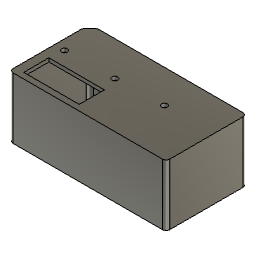
Waterproofing case - PLA case (Autodesk Fusion 360 design; units mm, degrees)
Autodesk Fusion 360 part; units mm, degrees
sketch "Sketch1" plane through (0, 0, 0) normal (0, 0, 1) x (1, 0, 0)
  line L0 (0, 0) -> (104, 0)
  line L1 (104, 0) -> (104, 51)
  line L2 (104, 51) -> (0, 51)
  line L3 (0, 51) -> (0, 0)
  dimension "d1" = 51
  dimension "d2" = 104
  constraint horizontal L0
  constraint vertical L1
  constraint horizontal L2
  constraint vertical L3
  constraint coincident L0.start L3.end
  measures "d1" distance of L0.start L2.end
  measures "d2" distance of L0.start L0.end
extrude "Extrude1" add sketch "Sketch1" along normal blind 2.5
sketch "Sketch2" plane through (0, 0, 2.5) normal (0, 0, 1) x (-1, 0, 0)
  line L0 (0, -51) -> (0, 0)
  line L1 (0, 0) -> (-104, 0)
  line L2 (-104, 0) -> (-104, -51)
  line L3 (-104, -51) -> (0, -51)
  line L4 (2.5, -53.5) -> (-106.5, -53.5)
  line L5 (-106.5, -53.5) -> (-106.5, 2.5)
  line L6 (-106.5, 2.5) -> (2.5, 2.5)
  line L7 (2.5, 2.5) -> (2.5, -53.5)
  dimension "d5" = 2.5
  dimension "d6" = 2.5
  dimension "d7" = 2.5
  dimension "d8" = 2.5
  constraint horizontal L4
  constraint vertical L5
  constraint horizontal L6
  constraint vertical L7
  measures "d5" distance of L1 L6
  measures "d6" distance of L2 L5
  measures "d7" distance of L3 L4
  measures "d8" distance of L0 L7
extrude "Extrude2" add sketch "Sketch2" against normal blind 42.5
fillet "Fillet1" radius 2.5 8 edges at (-2.5, -2.5, -18.75) (106.5, -2.5, -18.75) (106.5, 53.5, -18.75) (0, 0, -20) (-2.5, 53.5, -18.75) (0, 51, -20) (104, 0, -20) (104, 51, -20)
sketch "Sketch3" plane through (0, 0, 0) normal (0, 0, 1) x (1, 0, 0)
  line L0 (100, 19) -> (61.43, 19)
  line L1 (61.43, 19) -> (61.43, 1.5)
  line L2 (61.43, 1.5) -> (100, 1.5)
  line L3 (100, 1.5) -> (100, 19)
  line L4 (2.5, 0) -> (101.5, 0)
  line L5 (104, 2.5) -> (104, 48.5)
  circle A0 centre (97.5, 28.9) radius 2
  circle A1 centre (64.005, 29.5) radius 2
  circle A2 centre (29.495, 30.5) radius 2
  line L6 (106.5, 51) -> (106.5, 0)
  dimension "d13" = 38.57
  dimension "d14" = 17.5
  dimension "d15" = 1.5
  dimension "d16" = 4
  dimension "d17" = 4
  dimension "d18" = 4
  dimension "d19" = 4
  dimension "d20" = 9
  dimension "d21" = 9.9
  dimension "d22" = 10.5
  dimension "d23" = 11.5
  dimension "d24" = 33.495
  dimension "d25" = 34.51
  constraint horizontal L0
  constraint vertical L1
  constraint horizontal L2
  constraint vertical L3
  measures "d13" distance of L0.start L0.end
  measures "d14" distance of L0.start L2.end
  measures "d15" distance of L2 L4
  measures "d16" distance of L3 L5
  measures "d17" diameter of A0
  measures "d18" diameter of A1
  measures "d19" diameter of A2
  measures "d20" distance of A0.centre L6
  measures "d21" distance of L0 A0.centre
  measures "d22" distance of L0 A1.centre
  measures "d23" distance of L0 A2.centre
  measures "d24" horizontal distance of A0.centre A1.centre
  measures "d25" horizontal distance of A1.centre A2.centre
sketch "Sketch7" plane through (0, 0, 2.5) normal (0, 0, 1) x (-1, 0, 0)
  arc A0 (0, -53.5) -> (2.5, -51) centre (0, -51) ccw
  line L0 (2.5, -51) -> (2.5, 0)
  arc A1 (2.5, 0) -> (0, 2.5) centre (0, 0) ccw
  line L1 (0, 2.5) -> (-104, 2.5)
  arc A2 (-104, 2.5) -> (-106.5, 0) centre (-104, 0) ccw
  line L2 (-106.5, 0) -> (-106.5, -51)
  arc A3 (-106.5, -51) -> (-104, -53.5) centre (-104, -51) ccw
  line L3 (-104, -53.5) -> (0, -53.5)
  line L4 (-3.5, -19) -> (-42.07, -19)
  line L5 (-42.07, -19) -> (-42.07, -1.5)
  line L6 (-42.07, -1.5) -> (-3.5, -1.5)
  line L7 (-3.5, -1.5) -> (-3.5, -19)
  circle A4 centre (-6.5, -28.9) radius 2
  circle A5 centre (-41.01, -29.5) radius 2
  circle A6 centre (-74.505, -30.5) radius 2
  dimension "d49" = 38.57
  dimension "d50" = 17.5
  dimension "d51" = 4
  dimension "d52" = 6
  dimension "d53" = 4
  dimension "d54" = 4
  dimension "d55" = 4
  dimension "d56" = 9.9
  dimension "d57" = 10.5
  dimension "d58" = 11.5
  dimension "d59" = 9
  dimension "d60" = 34.51
  dimension "d61" = 33.495
  constraint horizontal L4
  constraint vertical L5
  constraint horizontal L6
  constraint vertical L7
  measures "d49" distance of L4.start L4.end
  measures "d50" distance of L4.start L6.end
  measures "d51" distance of L1 L6
  measures "d52" distance of L0 L7
  measures "d53" diameter of A4
  measures "d54" diameter of A5
  measures "d55" diameter of A6
  measures "d56" distance of L4 A4.centre
  measures "d57" distance of L4 A5.centre
  measures "d58" distance of L4 A6.centre
  measures "d59" distance of L0 A4.centre
  measures "d60" horizontal distance of A4.centre A5.centre
  measures "d61" horizontal distance of A5.centre A6.centre
extrude "Extrude6" cut sketch "Sketch7" against normal blind 50 contours L4 L5 L6 L7 | A4 | A5 | A6
sketch "Sketch8" plane through (0, 0, 0) normal (0, 0, 1) x (1, 0, 0)
sketch "Sketch9" plane through (0, 0, 0) normal (0, 0, -1) x (1, 0, 0)
  circle A0 centre (6.5, -28.9) radius 2
  line L0 (42.07, -1.5) -> (42.07, -19)
  line L1 (42.07, -19) -> (3.5, -19)
  line L2 (3.5, -19) -> (3.5, -1.5)
  line L3 (3.5, -1.5) -> (42.07, -1.5)
  circle A1 centre (41.01, -29.5) radius 2
  circle A2 centre (74.505, -30.5) radius 2
  arc A3 (101.5, -51) -> (104, -48.5) centre (101.5, -48.5) ccw
  line L4 (104, -48.5) -> (104, -2.5)
  arc A4 (104, -2.5) -> (101.5, 0) centre (101.5, -2.5) ccw
  line L5 (101.5, 0) -> (2.5, 0)
  arc A5 (2.5, 0) -> (0, -2.5) centre (2.5, -2.5) ccw
  line L6 (0, -2.5) -> (0, -48.5)
  arc A6 (0, -48.5) -> (2.5, -51) centre (2.5, -48.5) ccw
  line L7 (2.5, -51) -> (101.5, -51)
extrude "Extrude7" add sketch "Sketch9" against normal blind 2.5 contours A0 | A1 | A2
sketch "Sketch10" plane through (0, 0, 0) normal (0, 0, -1) x (1, 0, 0)
  line L0 (42.07, -1.5) -> (42.07, -19)
  line L1 (42.07, -19) -> (3.5, -19)
  line L2 (3.5, -19) -> (3.5, -1.5)
  line L3 (3.5, -1.5) -> (42.07, -1.5)
  arc A0 (101.5, -51) -> (104, -48.5) centre (101.5, -48.5) ccw
  line L4 (104, -48.5) -> (104, -2.5)
  arc A1 (104, -2.5) -> (101.5, 0) centre (101.5, -2.5) ccw
  line L5 (101.5, 0) -> (2.5, 0)
  arc A2 (2.5, 0) -> (0, -2.5) centre (2.5, -2.5) ccw
  line L6 (0, -2.5) -> (0, -48.5)
  arc A3 (0, -48.5) -> (2.5, -51) centre (2.5, -48.5) ccw
  line L7 (2.5, -51) -> (101.5, -51)
  circle A4 centre (4.4, -28.9) radius 2
  circle A5 centre (38.91, -29.5) radius 2
  circle A6 centre (72.405, -30.5) radius 2
  line L8 (0, -48.5) -> (0, -2.5)
  dimension "d66" = 4
  dimension "d67" = 4
  dimension "d68" = 4
  dimension "d69" = 4.4
  dimension "d70" = 38.91
  dimension "d71" = 72.405
  dimension "d72" = 9.9
  dimension "d73" = 10.5
  dimension "d74" = 11.5
  measures "d66" diameter of A4
  measures "d67" diameter of A5
  measures "d68" diameter of A6
  measures "d69" distance of A4.centre L8
  measures "d70" distance of A5.centre L8
  measures "d71" distance of A6.centre L8
  measures "d72" distance of L1 A4.centre
  measures "d73" distance of L1 A5.centre
  measures "d74" distance of L1 A6.centre
extrude "Extrude8" cut sketch "Sketch10" against normal blind 15 contours A4 | A5 | A6
sketch "Sketch11" plane through (0, 0, -40) normal (0, 0, -1) x (1, 0, 0)
  arc A0 (-2.5, -51) -> (0, -53.5) centre (0, -51) ccw
  line L0 (0, -53.5) -> (104, -53.5)
  arc A1 (104, -53.5) -> (106.5, -51) centre (104, -51) ccw
  line L1 (106.5, -51) -> (106.5, 0)
  arc A2 (106.5, 0) -> (104, 2.5) centre (104, 0) ccw
  line L2 (104, 2.5) -> (0, 2.5)
  arc A3 (0, 2.5) -> (-2.5, 0) centre (0, 0) ccw
  line L3 (-2.5, 0) -> (-2.5, -51)
  line L4 (101.5, -51) -> (2.5, -51)
  arc A4 (0, -48.5) -> (2.5, -51) centre (2.5, -48.5) ccw
  line L5 (0, -48.5) -> (0, -2.5)
  arc A5 (2.5, 0) -> (0, -2.5) centre (2.5, -2.5) ccw
  line L6 (2.5, 0) -> (101.5, 0)
  arc A6 (104, -2.5) -> (101.5, 0) centre (101.5, -2.5) ccw
  line L7 (104, -2.5) -> (104, -48.5)
  arc A7 (101.5, -51) -> (104, -48.5) centre (101.5, -48.5) ccw
  line L8 (0, -53.5) -> (-2.5, -51)
  constraint coincident A0.end L0.start
  constraint coincident A0.start L3.end
sketch "Sketch12" plane through (0, 0, -40) normal (0, 0, -1) x (1, 0, 0)
  arc A0 (-2.5, -51) -> (0, -53.5) centre (0, -51) ccw
  line L0 (0, -53.5) -> (104, -53.5)
  arc A1 (104, -53.5) -> (106.5, -51) centre (104, -51) ccw
  line L1 (106.5, -51) -> (106.5, 0)
  arc A2 (106.5, 0) -> (104, 2.5) centre (104, 0) ccw
  line L2 (104, 2.5) -> (0, 2.5)
  arc A3 (0, 2.5) -> (-2.5, 0) centre (0, 0) ccw
  line L3 (-2.5, 0) -> (-2.5, -51)
  line L4 (101.5, -51) -> (2.5, -51)
  arc A4 (0, -48.5) -> (2.5, -51) centre (2.5, -48.5) ccw
  line L5 (0, -48.5) -> (0, -2.5)
  arc A5 (2.5, 0) -> (0, -2.5) centre (2.5, -2.5) ccw
  line L6 (2.5, 0) -> (101.5, 0)
  arc A6 (104, -2.5) -> (101.5, 0) centre (101.5, -2.5) ccw
  line L7 (104, -2.5) -> (104, -48.5)
  arc A7 (101.5, -51) -> (104, -48.5) centre (101.5, -48.5) ccw
  line L8 (0, -53.5) -> (-2.5731, -53.5)
  line L9 (-2.5731, -53.5) -> (-2.5, -51)
  constraint coincident A0.end L0.start
  constraint tangent A0 L8
  constraint coincident A0.start L3.end
sketch "Sketch13" plane through (0, 0, -40) normal (0, 0, -1) x (1, 0, 0)
  arc A0 (-2.5, -51) -> (0, -53.5) centre (0, -51) ccw
  line L0 (0, -53.5) -> (104, -53.5)
  arc A1 (104, -53.5) -> (106.5, -51) centre (104, -51) ccw
  line L1 (106.5, -51) -> (106.5, 0)
  arc A2 (106.5, 0) -> (104, 2.5) centre (104, 0) ccw
  line L2 (104, 2.5) -> (0, 2.5)
  arc A3 (0, 2.5) -> (-2.5, 0) centre (0, 0) ccw
  line L3 (-2.5, 0) -> (-2.5, -51)
  line L4 (101.5, -51) -> (2.5, -51)
  arc A4 (0, -48.5) -> (2.5, -51) centre (2.5, -48.5) ccw
  line L5 (0, -48.5) -> (0, -2.5)
  arc A5 (2.5, 0) -> (0, -2.5) centre (2.5, -2.5) ccw
  line L6 (2.5, 0) -> (101.5, 0)
  arc A6 (104, -2.5) -> (101.5, 0) centre (101.5, -2.5) ccw
  line L7 (104, -2.5) -> (104, -48.5)
  arc A7 (101.5, -51) -> (104, -48.5) centre (101.5, -48.5) ccw
sketch "Sketch14" plane through (0, 0, -40) normal (0, 0, -1) x (1, 0, 0)
  arc A0 (-2.5, -51) -> (0, -53.5) centre (0, -51) ccw
  line L0 (0, -53.5) -> (104, -53.5)
  arc A1 (104, -53.5) -> (106.5, -51) centre (104, -51) ccw
  line L1 (106.5, -51) -> (106.5, 0)
  arc A2 (106.5, 0) -> (104, 2.5) centre (104, 0) ccw
  line L2 (104, 2.5) -> (0, 2.5)
  arc A3 (0, 2.5) -> (-2.5, 0) centre (0, 0) ccw
  line L3 (-2.5, 0) -> (-2.5, -51)
  line L4 (101.5, -51) -> (2.5, -51)
  arc A4 (0, -48.5) -> (2.5, -51) centre (2.5, -48.5) ccw
  line L5 (0, -48.5) -> (0, -2.5)
  arc A5 (2.5, 0) -> (0, -2.5) centre (2.5, -2.5) ccw
  line L6 (2.5, 0) -> (101.5, 0)
  arc A6 (104, -2.5) -> (101.5, 0) centre (101.5, -2.5) ccw
  line L7 (104, -2.5) -> (104, -48.5)
  arc A7 (101.5, -51) -> (104, -48.5) centre (101.5, -48.5) ccw
  line L8 (2.5821, -53.5) -> (-2.5, -48.4298)
  line L9 (2.5821, -53.5) -> (-3.6803, -53.5)
  line L10 (-3.6803, -53.5) -> (-2.5, -48.4298)
  constraint coincident L0 L8.start
  constraint coincident L3 L8.end
  constraint perpendicular L3 L9
extrude "Extrude9" cut sketch "Sketch14" against normal blind 49 contours A0 L0 L3 L8 L9
fillet "Fillet2" radius 3 2 edges at (2.5821, 53.5, -18.75) (-2.5, 48.4298, -18.75)
sketch "Sketch6" plane through (0, 0, 2.5) normal (0, 0, 1) x (-1, 0, 0)
  arc A0 (0, -53.5) -> (2.5, -51) centre (0, -51) ccw
  line L0 (2.5, -51) -> (2.5, 0)
  arc A1 (2.5, 0) -> (0, 2.5) centre (0, 0) ccw
  line L1 (0, 2.5) -> (-104, 2.5)
  arc A2 (-104, 2.5) -> (-106.5, 0) centre (-104, 0) ccw
  line L2 (-106.5, 0) -> (-106.5, -51)
  arc A3 (-106.5, -51) -> (-104, -53.5) centre (-104, -51) ccw
  line L3 (-104, -53.5) -> (0, -53.5)
  line L4 (-3.5, -19) -> (-42.07, -19)
  line L5 (-42.07, -19) -> (-42.07, -1.5)
  line L6 (-42.07, -1.5) -> (-3.5, -1.5)
  line L7 (-3.5, -1.5) -> (-3.5, -19)
  circle A4 centre (-6.5, -28.9) radius 2
  circle A5 centre (-39.995, -29.5) radius 2
  circle A6 centre (-74.505, -30.5) radius 2
  dimension "d34" = 38.57
  dimension "d35" = 17.5
  dimension "d36" = 6
  dimension "d37" = 4
  dimension "d38" = 4
  dimension "d39" = 4
  dimension "d40" = 4
  dimension "d41" = 9.9
  dimension "d42" = 10.5
  dimension "d43" = 11.5
  dimension "d44" = 9
  dimension "d45" = 33.495
  dimension "d46" = 34.51
  constraint horizontal L4
  constraint vertical L5
  constraint horizontal L6
  constraint vertical L7
  measures "d34" distance of L4.start L4.end
  measures "d35" distance of L4.start L6.end
  measures "d36" distance of L0 L7
  measures "d37" distance of L1 L6
  measures "d38" diameter of A4
  measures "d39" diameter of A5
  measures "d40" diameter of A6
  measures "d41" distance of L4 A4.centre
  measures "d42" distance of L4 A5.centre
  measures "d43" distance of L4 A6.centre
  measures "d44" distance of L0 A4.centre
  measures "d45" horizontal distance of A4.centre A5.centre
  measures "d46" horizontal distance of A5.centre A6.centre
extrude "Extrude5" [suppressed]
extrude "Extrude3" [suppressed]
extrude "Extrude4" [suppressed]
sketch "Sketch4" plane through (0, 0, 0) normal (0, 0, 1) x (1, 0, 0)
sketch "Sketch5" plane through (0, 0, 0) normal (0, 0, 1) x (1, 0, 0)
  line L0 (104, 51) -> (0, 51)
  line L1 (0, 51) -> (0, 0)
  line L2 (0, 0) -> (104, 0)
  line L3 (104, 0) -> (104, 51)
  line L4 (0, -2.5) -> (104, -2.5)
  line L5 (106.5, 0) -> (106.5, 51)
  dimension "d30" = 104
  dimension "d31" = 51
  dimension "d32" = 2.5
  dimension "d33" = 2.5
  constraint horizontal L0
  constraint vertical L1
  constraint horizontal L2
  constraint vertical L3
  measures "d30" distance of L0.start L0.end
  measures "d31" distance of L0.start L2.end
  measures "d32" distance of L2 L4
  measures "d33" distance of L3 L5
